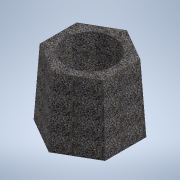
# Autodesk Inventor part: smietnik1
Saved by Autodesk Inventor 2021 (Build 250183000, 183)
## iProperties
Created: 2025-11-29
Part Number: smietnik1
Material: Concrete
Document SubType Name: Modeling
Designer: huber
Density: 2.40731 g/cm^3
Appearance: Coarse - White
Author: huber
Autodesk Inventor part; units mm, degrees
ref_plane "YZ Plane" through (0, 0, 0) normal (1, 0, 0) x (0, 1, 0)
ref_plane "XY Plane" through (0, 0, 0) normal (0, 0, 1) x (1, 0, 0)
sketch "Sketch1" plane through (0, 0, 0) normal (0, 1, 0) x (-1, 0, 0)
  line L0 (0, -433.0127) -> (-375, -216.5064)
  line L1 (-375, -216.5064) -> (-375, 216.5064)
  line L2 (-375, 216.5064) -> (0, 433.0127)
  line L3 (0, 433.0127) -> (375, 216.5064)
  line L4 (375, 216.5064) -> (375, -216.5064)
  line L5 (375, -216.5064) -> (0, -433.0127)
  line L6 (0, -606.2178) -> (0, 606.2178) projected
  point P0 (0, 0)
  point P1 (0, 0)
  dimension "d0" = 750
  constraints: 12 end point, 1 coincident, 1 point on line, 13 other
  measures "d0" distance between parallel lines of L1 L4
ref_plane "Work Plane1" through (0, 700, 0) normal (0, 1, 0) x (-1, 0, 0)
sketch "Sketch2" plane through (0, 700, 0) normal (0, 1, 0) x (-1, 0, 0)
  line L0 (0, -386.8247) -> (-335, -193.4123)
  line L1 (-335, -193.4123) -> (-335, 193.4123)
  line L2 (-335, 193.4123) -> (0, 386.8247)
  line L3 (0, 386.8247) -> (335, 193.4123)
  line L4 (335, 193.4123) -> (335, -193.4123)
  line L5 (335, -193.4123) -> (0, -386.8247)
  point P0 (0, 0)
  point P1 (0, 0)
  dimension "d2" = 670
  constraints: 12 end point, 1 coincident, 1 vertical, 13 other
  measures "d2" distance between parallel lines of L1 L4
loft "Loft1" add profiles "Sketch1", "Sketch2"
sketch "Sketch3" plane through (335, 700, 193.4123) normal (0, 1, 0) x (1, 0, 0)
  circle A0 centre (-335, 193.4123) radius 255
  dimension "d7" = 510
  constraints: 1 centre point, 1 coincident
  measures "d7" diameter of A0
extrude "Extrusion1" cut sketch "Sketch3" against normal blind 620
body "Solid1"
